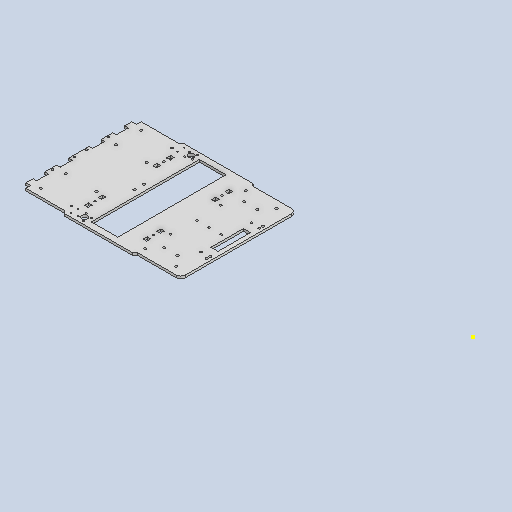
# Autodesk Inventor part: нижняя пластина
Saved by Autodesk Inventor 2024.2 (Build 282272000, 272)
## iProperties
Created: 2025-11-23
Part Number: нижняя пластина
Material: Типовые
Document SubType Name: Modeling
Designer: katya_notebook
Density: 1 g/cm^3
Appearance: По умолчанию
Author: katya_notebook
Autodesk Inventor part; units mm, degrees
ref_plane "YZ Plane" through (0, 0, 0) normal (1, 0, 0) x (0, 1, 0)
ref_plane "XZ Plane" through (0, 0, 0) normal (0, 1, 0) x (-1, 0, 0)
ref_plane "XY Plane" through (0, 0, 0) normal (0, 0, 1) x (1, 0, 0)
ref_plane "РабПлоскость1" through (-553.278877, -264.300199, 1.422232) normal (0, 1, 0) x (-1, 0, 0)
sketch "Эскиз1" plane through (-553.278877, -264.300199, 1.422232) normal (0, 1, 0) x (-1, 0, 0)
  line L0 (-30, 163.500004) -> (30, 163.500003)
  line L1 (-30, -31.5) -> (30, -31.5)
  line L2 (46.476267, 163.500003) -> (-223.523733, 163.500003)
  line L3 (-223.523733, 163.500003) -> (-223.523733, -31.5)
  line L4 (-223.523733, -31.5) -> (46.476267, -31.5)
  line L5 (46.476267, -31.5) -> (46.476267, 163.500003)
  point P0 (-553.278877, -1.422232)
  point P1 (-30, -30)
  point P2 (30, -30)
  point P3 (30, 162.000003)
  point P4 (-30, 162.000004)
  dimension "d1" = 270
  dimension "d6" = 0
  dimension "d7" = 0
  constraints: 8 end point, 2 coincident, 2 parallel, 1 horizontal, 1 perpendicular
  measures "d1" distance of L2.start L2.end
  measures "d6" distance from line of L4 L1.end
  measures "d7" distance from line of L2 L0.end
extrude "Выдавливание1" add sketch "Эскиз1" along normal blind 4
sketch "Эскиз2" plane through (-553.278877, -264.300199, 1.422232) normal (0, -1, 0) x (1, 0, 0)
  circle A0 centre (26, 108.500004) radius 2
  circle A1 centre (-26, 151.000003) radius 2
  circle A2 centre (26, 151.000004) radius 2
  circle A3 centre (-26, 108.500003) radius 2
  line L0 (-21.5, 122.000003) -> (-21.5, 157.000003)
  line L1 (-23.5, 122.000003) -> (-21.5, 122.000003)
  line L2 (-23.5, 157.000003) -> (-23.5, 122.000003)
  line L3 (-30, 157.000003) -> (-23.5, 157.000003)
  line L4 (-30, 157.000003) -> (-30, 103.500003)
  line L5 (-30, 103.500003) -> (30, 103.500004)
  line L6 (30, 103.500004) -> (30, 157.000004)
  line L7 (23.5, 157.000004) -> (30, 157.000004)
  line L8 (23.5, 122.000004) -> (23.5, 157.000004)
  line L9 (21.5, 122.000004) -> (23.5, 122.000004)
  line L10 (21.5, 157.000004) -> (21.5, 122.000004)
  line L11 (-21.5, 157.000003) -> (21.5, 157.000004)
  circle A4 centre (26, 23.5) radius 2
  circle A5 centre (-26, -19) radius 2
  circle A6 centre (26, -19) radius 2
  circle A7 centre (-26, 23.5) radius 2
  line L12 (-21.5, 10) -> (-21.5, -25)
  line L13 (-21.5, -25) -> (21.5, -25)
  line L14 (21.5, -25) -> (21.5, 10)
  line L15 (21.5, 10) -> (23.5, 10)
  line L16 (23.5, 10) -> (23.5, -25)
  line L17 (23.5, -25) -> (30, -25)
  line L18 (30, 28.5) -> (30, -25)
  line L19 (-30, 28.5) -> (30, 28.5)
  line L20 (-30, -25) -> (-30, 28.5)
  line L21 (-30, -25) -> (-23.5, -25)
  line L22 (-23.5, -25) -> (-23.5, 10)
  line L23 (-23.5, 10) -> (-21.5, 10)
  circle A8 centre (26, -19) radius 2
  circle A9 centre (26, 23.5) radius 2
  circle A10 centre (-26, -19) radius 2
  circle A11 centre (-26, 23.5) radius 2
  circle A12 centre (26, 108.500004) radius 2
  circle A13 centre (26, 151.000004) radius 2
  circle A14 centre (-26, 108.500003) radius 2
  circle A15 centre (-26, 151.000003) radius 2
  point P0 (553.278877, -1.422232)
  constraints: 8 centre point, 8 coincident, 8 concentric
extrude "Выдавливание2" cut sketch "Эскиз2" against normal blind 4 contours A0 | A1 | A2 | A3 | A4 | A5 | A6 | A7
sketch "Эскиз3" plane through (-553.278877, -264.300199, 1.422232) normal (0, -1, 0) x (1, 0, 0)
  spline S0 degree 3 poles (167.530647, -1.5) (167.530647, -1.675228) (167.505938, -1.863112) (167.406969, -2.216269) (167.332996, -2.381628) (167.143154, -2.701977) (167.002629, -2.869355) (166.694843, -3.139058) (166.528045, -3.241917) (165.99333, -3.490366) (165.589204, -3.533982) (164.848659, -3.417135) (164.512124, -3.257434) (164.024214, -2.845742) (163.799855, -2.568258) (163.628417, -2.126382) (163.592902, -2.011125) (163.543842, -1.762124) (163.530647, -1.627897) (163.530647, -1.372102) (163.543842, -1.237875) (163.592902, -0.988874) (163.628417, -0.873617) (163.799855, -0.431742) (164.024214, -0.154257) (164.512124, 0.257435) (164.848659, 0.417136) (165.589204, 0.533983) (165.99333, 0.490367) (166.528045, 0.241918) (166.694843, 0.139059) (167.002629, -0.130644) (167.143154, -0.298022) (167.332996, -0.618371) (167.406969, -0.78373) (167.505938, -1.136887) (167.530647, -1.324772) (167.530647, -1.5) knots -1.5971811 -1.5971811 -1.5971811 -1.5971811 -1.5446127 -1.5446127 -1.49204429 -1.49204429 -1.42257961 -1.42257961 -1.35311492 -1.35311492 -1.18239978 -1.18239978 -1.01168465 -1.01168465 -0.87532923 -0.87532923 -0.83695989 -0.83695989 -0.79859055 -0.79859055 -0.76022121 -0.76022121 -0.72185188 -0.72185188 -0.58549645 -0.58549645 -0.41478132 -0.41478132 -0.24406618 -0.24406618 -0.17460149 -0.17460149 -0.10513681 -0.10513681 -0.0525684 -0.0525684 0 0 0 0
  spline S1 degree 3 poles (190.047468, -1.5) (190.047468, -1.620288) (190.036518, -1.738724) (189.995823, -1.966144) (189.966063, -2.075131) (189.855778, -2.381563) (189.753425, -2.558671) (189.3863, -3.048352) (189.043184, -3.281704) (188.267032, -3.529213) (187.832995, -3.536652) (187.236348, -3.337829) (187.042108, -3.243447) (186.680736, -2.977295) (186.514082, -2.804962) (186.286366, -2.464282) (186.197167, -2.285548) (186.077558, -1.900195) (186.047468, -1.693486) (186.047468, -1.306513) (186.077558, -1.099804) (186.197167, -0.714451) (186.286366, -0.535718) (186.514082, -0.195037) (186.680736, -0.022705) (187.042108, 0.243448) (187.236348, 0.33783) (187.832995, 0.536653) (188.267032, 0.529214) (189.043184, 0.281704) (189.3863, 0.048353) (189.753425, -0.441328) (189.855778, -0.618437) (189.966063, -0.924868) (189.995823, -1.033855) (190.036518, -1.261275) (190.047468, -1.379712) (190.047468, -1.5) knots -1.53992103 -1.53992103 -1.53992103 -1.53992103 -1.50383465 -1.50383465 -1.46774826 -1.46774826 -1.39557548 -1.39557548 -1.21717391 -1.21717391 -1.03877234 -1.03877234 -0.96241242 -0.96241242 -0.88605249 -0.88605249 -0.8280065 -0.8280065 -0.76996052 -0.76996052 -0.71191453 -0.71191453 -0.65386854 -0.65386854 -0.57750862 -0.57750862 -0.50114869 -0.50114869 -0.32274712 -0.32274712 -0.14434556 -0.14434556 -0.07217278 -0.07217278 -0.03608639 -0.03608639 0 0 0 0
  circle A0 centre (203.047466, 23.5) radius 2
  circle A1 centre (203.047467, -19) radius 2
  circle A2 centre (151.047466, 23.5) radius 2
  circle A3 centre (151.047467, -19) radius 2
  line L0 (206.802962, 28.5) -> (146.802962, 28.5)
  line L1 (146.802962, 28.5) -> (146.802962, -22)
  line L2 (206.802962, -22) -> (206.802962, 28.5)
  line L3 (206.802962, -22) -> (146.802962, -22)
  point P0 (553.278877, -1.422232)
  point P1 (167.530647, -1.5)
  point P2 (190.047468, -1.5)
extrude "Выдавливание3" cut sketch "Эскиз3" against normal blind 10 contours S0 | S1 | A0 | A1 | A2 | A3
sketch "Эскиз4" plane through (-553.278877, -264.300199, 1.422232) normal (0, -1, 0) x (1, 0, 0)
  circle A0 centre (151.047466, 108.500004) radius 2
  circle A1 centre (203.047466, 108.500003) radius 2
  spline S0 degree 3 poles (190.047468, 133.500003) (190.047468, 133.620291) (190.036518, 133.738728) (189.995823, 133.966148) (189.966063, 134.075135) (189.855778, 134.381566) (189.753425, 134.558675) (189.3863, 135.048356) (189.043184, 135.281707) (188.267032, 135.529217) (187.832995, 135.536656) (187.236348, 135.337833) (187.042108, 135.243451) (186.680736, 134.977298) (186.514082, 134.804966) (186.286366, 134.464285) (186.197167, 134.285552) (186.077558, 133.900199) (186.047468, 133.69349) (186.047468, 133.306517) (186.077558, 133.099808) (186.197167, 132.714455) (186.286366, 132.535721) (186.514082, 132.195041) (186.680736, 132.022708) (187.042108, 131.756556) (187.236348, 131.662174) (187.832995, 131.46335) (188.267032, 131.47079) (189.043184, 131.718299) (189.3863, 131.95165) (189.753425, 132.441332) (189.855778, 132.61844) (189.966063, 132.924872) (189.995823, 133.033859) (190.036518, 133.261279) (190.047468, 133.379715) (190.047468, 133.500003) knots 0 0 0 0 0.03608639 0.03608639 0.07217278 0.07217278 0.14434556 0.14434556 0.32274712 0.32274712 0.50114869 0.50114869 0.57750862 0.57750862 0.65386854 0.65386854 0.71191453 0.71191453 0.76996052 0.76996052 0.8280065 0.8280065 0.88605249 0.88605249 0.96241242 0.96241242 1.03877234 1.03877234 1.21717391 1.21717391 1.39557548 1.39557548 1.46774826 1.46774826 1.50383465 1.50383465 1.53992103 1.53992103 1.53992103 1.53992103
  spline S1 degree 3 poles (167.530647, 133.500003) (167.530647, 133.675231) (167.505938, 133.863116) (167.406969, 134.216273) (167.332996, 134.381632) (167.143154, 134.701981) (167.002629, 134.869359) (166.694843, 135.139062) (166.528045, 135.241921) (165.99333, 135.49037) (165.589204, 135.533986) (164.848659, 135.417139) (164.512124, 135.257438) (164.024214, 134.845746) (163.799855, 134.568261) (163.628417, 134.126386) (163.592902, 134.011129) (163.543842, 133.762128) (163.530647, 133.627901) (163.530647, 133.372105) (163.543842, 133.237879) (163.592902, 132.988878) (163.628417, 132.873621) (163.799855, 132.431745) (164.024214, 132.154261) (164.512124, 131.742569) (164.848659, 131.582868) (165.589204, 131.466021) (165.99333, 131.509637) (166.528045, 131.758086) (166.694843, 131.860945) (167.002629, 132.130648) (167.143154, 132.298026) (167.332996, 132.618375) (167.406969, 132.783734) (167.505938, 133.136891) (167.530647, 133.324775) (167.530647, 133.500003) knots 0 0 0 0 0.0525684 0.0525684 0.10513681 0.10513681 0.17460149 0.17460149 0.24406618 0.24406618 0.41478132 0.41478132 0.58549645 0.58549645 0.72185188 0.72185188 0.76022121 0.76022121 0.79859055 0.79859055 0.83695989 0.83695989 0.87532923 0.87532923 1.01168465 1.01168465 1.18239978 1.18239978 1.35311492 1.35311492 1.42257961 1.42257961 1.49204429 1.49204429 1.5446127 1.5446127 1.5971811 1.5971811 1.5971811 1.5971811
  circle A2 centre (151.047467, 151.000004) radius 2
  circle A3 centre (203.047467, 151.000003) radius 2
  point P0 (553.278877, -1.422232)
  point P1 (190.047468, 133.500003)
  point P2 (167.530647, 133.500003)
extrude "Выдавливание4" cut sketch "Эскиз4" against normal blind 10
sketch "Эскиз6" plane through (-553.278877, -264.300199, 1.422232) normal (0, -1, 0) x (1, 0, 0)
  circle A0 centre (53.523733, 156.000002) radius 5
  circle A1 centre (53.523733, 156.000002) radius 2.5
  circle A2 centre (53.523733, 156.000002) radius 5
  circle A3 centre (53.523733, -23.999998) radius 5
  circle A4 centre (53.523733, -23.999998) radius 5
  point P0 (553.278877, -1.422232)
  constraints: 2 centre point, 2 coincident, 2 concentric
extrude "Выдавливание6" cut sketch "Эскиз6" against normal blind 10 contours A0 | A1 | A3
sketch "Эскиз7" plane through (-553.278877, -264.300199, 1.422232) normal (0, -1, 0) x (1, 0, 0)
  line L0 (30, 103.500004) -> (30, 157.000004)
  line L1 (-46.476267, 163.500003) -> (223.523733, 163.500003)
  line L2 (30.270127, 167.770131) -> (146.697322, 167.770131)
  line L3 (146.802962, 163.500003) -> (146.802962, 157.000003)
  line L4 (146.802962, 167.770131) -> (146.697322, 167.770131)
  line L5 (146.802962, 163.500003) -> (30, 163.500003)
  line L6 (30.000003, 28.5) -> (30.000003, -25)
  line L7 (30.000003, -25) -> (30.000003, -31.5)
  line L8 (146.802962, -31.5) -> (146.802962, -25)
  line L9 (146.802962, -35.5) -> (30.000003, -35.5)
  line L10 (30.000003, -31.5) -> (146.802962, -31.5)
  line L11 (30, 163.500003) -> (26, 163.500003)
  arc A0 (26, 163.500003) -> (30.270127, 167.770131) centre (22.8966, 170.873531) ccw
  line L12 (146.802962, 163.500003) -> (150.802962, 163.500003)
  arc A1 (146.802962, 167.770131) -> (150.802962, 163.500003) centre (154.237087, 170.72543) ccw
  line L13 (30.000003, -31.5) -> (26.000003, -31.5)
  line L14 (223.523733, -31.5) -> (-46.476267, -31.5)
  arc A2 (30.000003, -35.5) -> (26.000003, -31.5) centre (22.7085, -38.791502) ccw
  line L15 (146.802962, -31.5) -> (150.802962, -31.5)
  arc A3 (150.802962, -31.5) -> (146.802962, -35.5) centre (154.094465, -38.791502) ccw
  point P0 (553.278877, -1.422232)
  dimension "d23" = 8
  dimension "d24" = 8
  dimension "d26" = 8
  dimension "d28" = 8
  constraints: 18 end point, 8 point on circle, 5 point on line, 4 centre point, 2 collinear, 1 parallel
  measures "d23" radius of A0
  measures "d24" radius of A1
  measures "d26" radius of A2
  measures "d28" radius of A3
extrude "Выдавливание7" add sketch "Эскиз7" against normal blind 4
sketch "Эскиз8" plane through (-553.278877, -264.300199, 1.422232) normal (0, -1, 0) x (1, 0, 0)
  circle A0 centre (57.777238, 162.775524) radius 1.5
  circle A1 centre (60.299256, 151.746498) radius 1.5
  circle A2 centre (49.270229, 149.22448) radius 1.5
  circle A3 centre (46.748211, 160.253506) radius 1.5
  circle A4 centre (57.777238, 162.775524) radius 1.5
  circle A5 centre (60.299256, 151.746498) radius 1.5
  circle A6 centre (49.270229, 149.22448) radius 1.5
  circle A7 centre (46.748211, 160.253506) radius 1.5
  circle A8 centre (60.299256, -19.746494) radius 1.5
  circle A9 centre (57.777238, -30.775521) radius 1.5
  circle A10 centre (46.748211, -28.253503) radius 1.5
  circle A11 centre (49.270229, -17.224476) radius 1.5
  circle A12 centre (49.270229, -17.224476) radius 1.5
  circle A13 centre (60.299256, -19.746494) radius 1.5
  circle A14 centre (57.777238, -30.775521) radius 1.5
  circle A15 centre (46.748211, -28.253503) radius 1.5
  point P0 (553.278877, -1.422232)
  constraints: 8 centre point, 8 coincident, 8 concentric
extrude "Выдавливание8" cut sketch "Эскиз8" against normal blind 4
sketch "Эскиз9" plane through (-553.278877, -264.300199, 1.422232) normal (0, -1, 0) x (1, 0, 0)
  line L0 (223.523733, 163.500003) -> (223.523733, -31.5)
  line L1 (-46.476267, -31.5) -> (-46.476267, 163.500003)
  line L2 (223.523733, 163.500003) -> (-46.476267, 163.500003)
  line L3 (-46.476267, 163.500003) -> (-46.476267, -31.5)
  line L4 (-46.476267, -31.5) -> (223.523733, -31.5)
  line L5 (223.523733, -31.5) -> (223.523733, 163.500003)
  line L6 (223.523733, 66.000002) -> (-46.476267, 66.000002)
  line L7 (88.523733, 163.500003) -> (88.523733, -31.5)
  line L8 (66.023733, -25.499998) -> (111.023733, -25.499998)
  line L9 (111.023733, -25.499998) -> (111.023733, 157.500002)
  line L10 (111.023733, 157.500002) -> (66.023733, 157.500002)
  line L11 (66.023733, 157.500002) -> (66.023733, -25.499998)
  line L12 (66.023733, -25.499998) -> (111.023733, 157.500002) construction
  line L13 (111.023733, -25.499998) -> (66.023733, 157.500002) construction
  point P0 (553.278877, -1.422232)
  point P1 (88.523733, 66.000002)
  dimension "d33" = 183
  dimension "d34" = 45
  constraints: 24 end point, 7 midpoint, 4 parallel, 2 horizontal, 2 perpendicular
  measures "d33" distance of L8.end L9.end
  measures "d34" distance of L9.end L10.end
extrude "Выдавливание9" cut sketch "Эскиз9" against normal blind 4 contours L9 L8 L7 L6 | L6 L7 L10 L9 | L7 L6 L11 L10 | L7 L8 L11 L6
sketch "Эскиз10" plane through (-553.278877, -264.300199, 1.422232) normal (0, -1, 0) x (1, 0, 0)
  line L0 (36.973733, 147.850002) -> (34.973733, 147.850002)
  line L1 (36.973733, 147.850002) -> (36.973733, 152.650002)
  line L2 (35.973733, 147.850002) -> (35.973733, 152.650002)
  line L3 (36.973733, 159.350002) -> (34.973733, 159.350002)
  line L4 (36.973733, 150.250002) -> (34.973733, 150.250002)
  line L5 (36.973733, 159.350002) -> (36.973733, 164.150002)
  line L6 (36.973733, 161.750002) -> (33.994288, 161.750002)
  line L7 (33.994288, 161.750002) -> (35.973733, 159.350002)
  line L8 (35.973733, 164.150002) -> (35.973733, 159.350002)
  circle A0 centre (35.973733, 161.750002) radius 1
  circle A1 centre (35.973733, 150.250002) radius 1
  point P0 (553.278877, -1.422232)
  point P1 (34.973733, 147.000002)
  point P2 (30, 163.500005)
  point P3 (34.973733, 161.750002)
  point P4 (35.973733, 162.750002)
  point P5 (35.973733, 161.750002)
  constraints: 18 end point, 4 midpoint, 4 perpendicular, 2 horizontal, 1 horizontal alignment, 6 other
extrude "Выдавливание10" cut sketch "Эскиз10" against normal blind 10 contours A1 L2 L4 | L4 L2 A1 | A1 L4 L2 | L4 A1 L2 | A0 L8 L6 | L6 L8 A0 | A0 L6 L8 | L6 A0 L8
sketch "Эскиз11" plane through (-553.278877, -264.300199, 1.422232) normal (0, -1, 0) x (1, 0, 0)
  arc A0 (34.973733, -29.749998) -> (36.973733, -29.749998) centre (35.973733, -29.749998) ccw
  arc A1 (36.973733, -29.749998) -> (34.973733, -29.749998) centre (35.973733, -29.749998) ccw
  arc A2 (34.973733, -18.249998) -> (36.973733, -18.249998) centre (35.973733, -18.249998) ccw
  arc A3 (36.973733, -18.249998) -> (34.973733, -18.249998) centre (35.973733, -18.249998) ccw
  point P0 (553.278877, -1.422232)
extrude "Выдавливание11" cut sketch "Эскиз11" against normal blind 10
sketch "Эскиз12" plane through (-553.278877, -264.300199, 1.422232) normal (0, -1, 0) x (1, 0, 0)
  circle A0 centre (55.548733, 57.85394) radius 2
  circle A1 centre (55.548733, 73.85394) radius 2
  point P0 (553.278877, -1.422232)
extrude "Выдавливание12" cut sketch "Эскиз12" against normal blind 10
sketch "Эскиз13" plane through (-553.278877, -264.300199, 1.422232) normal (0, -1, 0) x (1, 0, 0)
  point P0 (553.278877, -1.422232)
sketch "Эскиз14" plane through (-553.278877, -264.300199, 1.422232) normal (0, -1, 0) x (1, 0, 0)
  circle A0 centre (217.523733, 18.5) radius 2
  circle A1 centre (217.523733, 113.500003) radius 2
  line L0 (150.802962, 163.500003) -> (223.523733, 163.500003)
  line L1 (223.523733, -31.5) -> (150.802962, -31.5)
  line L2 (223.523733, 163.500003) -> (223.523733, -31.5)
  circle A2 centre (217.523733, 24.5) radius 2
  circle A3 centre (217.523733, 107.500003) radius 2
  point P0 (553.278877, -1.422232)
  dimension "d43" = 4
  dimension "d44" = 4
  dimension "d45" = 50
  dimension "d46" = 50
  dimension "d47" = 6
  dimension "d48" = 6
  dimension "d51" = 4
  dimension "d52" = 6
  dimension "d53" = 6
  dimension "d54" = 4
  dimension "d55" = 6
  dimension "d56" = 6
  constraints: 4 centre point
  measures "d43" diameter of A1
  measures "d44" diameter of A0
  measures "d45" distance from line of L0 A1.centre
  measures "d46" distance from line of L1 A0.centre
  measures "d47" distance from line of L2 A0.centre
  measures "d48" distance from line of L2 A1.centre
  measures "d51" diameter of A3
  measures "d52" distance of A1.centre A3.centre
  measures "d53" distance from line of L2 A3.centre
  measures "d54" diameter of A2
  measures "d55" distance from line of L2 A2.centre
  measures "d56" distance of A0.centre A2.centre
extrude "Выдавливание13" cut sketch "Эскиз14" against normal blind 10
sketch "Эскиз15" plane through (-553.278877, -264.300199, 1.422232) normal (0, -1, 0) x (1, 0, 0)
  line L0 (216.523733, 93.576493) -> (204.523733, 93.576493)
  line L1 (204.523733, 93.576493) -> (204.523733, 38.576493)
  line L2 (204.523733, 38.576493) -> (216.523733, 38.576493)
  line L3 (216.523733, 38.576493) -> (216.523733, 93.576493)
  line L4 (216.523733, 93.576493) -> (204.523733, 38.576493) construction
  line L5 (204.523733, 93.576493) -> (216.523733, 38.576493) construction
  line L6 (223.523733, 163.500003) -> (223.523733, -31.5)
  point P0 (553.278877, -1.422232)
  point P1 (210.523733, 66.076493)
  dimension "d57" = 13
  dimension "d58" = 12
  dimension "d59" = 55
  constraints: 12 end point, 2 midpoint, 2 parallel, 1 horizontal, 1 perpendicular
  measures "d57" distance from line of point (210.524, 66.076) L6
  measures "d58" distance of L0.start L0.end
  measures "d59" distance of L0.end L1.end
extrude "Выдавливание14" cut sketch "Эскиз15" against normal blind 10
sketch "Эскиз16" plane through (-553.278877, -264.300199, 1.422232) normal (0, -1, 0) x (1, 0, 0)
  spline S0 degree 3 poles (195.773733, 65.9) (195.773733, 66.088725) (195.735944, 66.289784) (195.582756, 66.659245) (195.467375, 66.827679) (195.201416, 67.093638) (195.03298, 67.209022) (194.663513, 67.362213) (194.462453, 67.4) (194.085014, 67.4) (193.883953, 67.362213) (193.514486, 67.209022) (193.346051, 67.093638) (193.080092, 66.827679) (192.964711, 66.659245) (192.811522, 66.289784) (192.773733, 66.088725) (192.773733, 65.711276) (192.811522, 65.510217) (192.964711, 65.140756) (193.080092, 64.972321) (193.346051, 64.706363) (193.514486, 64.590979) (193.883953, 64.437788) (194.085014, 64.4) (194.462453, 64.4) (194.663513, 64.437788) (195.03298, 64.590979) (195.201416, 64.706363) (195.467375, 64.972321) (195.582756, 65.140756) (195.735944, 65.510217) (195.773733, 65.711276) (195.773733, 65.9) knots -0.905867 -0.905867 -0.905867 -0.905867 -0.84924956 -0.84924956 -0.79263212 -0.79263212 -0.73601619 -0.73601619 -0.67940025 -0.67940025 -0.62278432 -0.62278432 -0.56616839 -0.56616839 -0.50955095 -0.50955095 -0.4529335 -0.4529335 -0.39631606 -0.39631606 -0.33969861 -0.33969861 -0.28308268 -0.28308268 -0.22646675 -0.22646675 -0.16985082 -0.16985082 -0.11323489 -0.11323489 -0.05661744 -0.05661744 0 0 0 0
  spline S1 degree 3 poles (172.273733, 66.1) (172.273733, 65.911276) (172.311522, 65.710217) (172.464711, 65.340756) (172.580092, 65.172321) (172.846051, 64.906363) (173.014486, 64.790979) (173.383953, 64.637788) (173.585014, 64.6) (173.962453, 64.6) (174.163513, 64.637788) (174.53298, 64.790979) (174.701416, 64.906363) (174.967375, 65.172321) (175.082756, 65.340756) (175.235944, 65.710217) (175.273733, 65.911276) (175.273733, 66.288725) (175.235944, 66.489784) (175.082756, 66.859245) (174.967375, 67.027679) (174.701416, 67.293638) (174.53298, 67.409022) (174.163513, 67.562213) (173.962453, 67.6) (173.585014, 67.6) (173.383953, 67.562213) (173.014486, 67.409022) (172.846051, 67.293638) (172.580092, 67.027679) (172.464711, 66.859245) (172.311522, 66.489784) (172.273733, 66.288725) (172.273733, 66.1) knots -0.905867 -0.905867 -0.905867 -0.905867 -0.84924956 -0.84924956 -0.79263212 -0.79263212 -0.73601619 -0.73601619 -0.67940025 -0.67940025 -0.62278432 -0.62278432 -0.56616839 -0.56616839 -0.50955095 -0.50955095 -0.4529335 -0.4529335 -0.39631606 -0.39631606 -0.33969861 -0.33969861 -0.28308268 -0.28308268 -0.22646675 -0.22646675 -0.16985082 -0.16985082 -0.11323489 -0.11323489 -0.05661744 -0.05661744 0 0 0 0
  spline S2 degree 3 poles (154.773733, 65.9) (154.773733, 66.088725) (154.735944, 66.289784) (154.582756, 66.659245) (154.467375, 66.827679) (154.201416, 67.093638) (154.03298, 67.209022) (153.663513, 67.362213) (153.462453, 67.4) (153.085014, 67.4) (152.883953, 67.362213) (152.514486, 67.209022) (152.346051, 67.093638) (152.080092, 66.827679) (151.964711, 66.659245) (151.811522, 66.289784) (151.773733, 66.088725) (151.773733, 65.711276) (151.811522, 65.510217) (151.964711, 65.140756) (152.080092, 64.972321) (152.346051, 64.706363) (152.514486, 64.590979) (152.883953, 64.437788) (153.085014, 64.4) (153.462453, 64.4) (153.663513, 64.437788) (154.03298, 64.590979) (154.201416, 64.706363) (154.467375, 64.972321) (154.582756, 65.140756) (154.735944, 65.510217) (154.773733, 65.711276) (154.773733, 65.9) knots -0.905867 -0.905867 -0.905867 -0.905867 -0.84924956 -0.84924956 -0.79263212 -0.79263212 -0.73601619 -0.73601619 -0.67940025 -0.67940025 -0.62278432 -0.62278432 -0.56616839 -0.56616839 -0.50955095 -0.50955095 -0.4529335 -0.4529335 -0.39631606 -0.39631606 -0.33969861 -0.33969861 -0.28308268 -0.28308268 -0.22646675 -0.22646675 -0.16985082 -0.16985082 -0.11323489 -0.11323489 -0.05661744 -0.05661744 0 0 0 0
  point P0 (553.278877, -1.422232)
  point P1 (195.773733, 65.9)
  point P2 (172.273733, 66.1)
  point P3 (154.773733, 65.9)
extrude "Выдавливание15" cut sketch "Эскиз16" against normal blind 10
sketch "Эскиз17" plane through (-553.278877, -260.300199, 1.422232) normal (0, 1, 0) x (1, 0, 0)
  line L0 (-46.476267, -143.500003) -> (-46.476267, -123.500003)
  line L1 (-46.476267, -143.500003) -> (-40.476267, -143.500003)
  line L2 (-40.476267, -123.500003) -> (-40.476267, -143.500003)
  line L3 (-46.476267, -123.500003) -> (-40.476267, -123.500003)
  line L4 (-46.476267, -103.500003) -> (-46.476267, -83.500003)
  line L5 (-46.476267, -103.500003) -> (-40.476267, -103.500003)
  line L6 (-40.476267, -83.500003) -> (-40.476267, -103.500003)
  line L7 (-46.476267, -83.500003) -> (-40.476267, -83.500003)
  line L8 (-46.476267, -48.5) -> (-46.476267, -28.5)
  line L9 (-46.476267, -48.5) -> (-40.476267, -48.5)
  line L10 (-40.476267, -28.5) -> (-40.476267, -48.5)
  line L11 (-46.476267, -28.5) -> (-40.476267, -28.5)
  line L12 (-46.476267, -8.5) -> (-46.476267, 11.5)
  line L13 (-46.476267, -8.5) -> (-40.476267, -8.5)
  line L14 (-40.476267, 11.5) -> (-40.476267, -8.5)
  line L15 (-46.476267, 11.5) -> (-40.476267, 11.5)
  circle A0 centre (-43.476267, -113.500003) radius 1.75
  circle A1 centre (-43.476267, -76.375003) radius 1.75
  circle A2 centre (-43.476267, -55.625003) radius 1.75
  circle A3 centre (-43.476267, -18.5) radius 1.75
  point P0 (553.278877, 1.422232)
extrude "Выдавливание16" cut sketch "Эскиз17" against normal blind 10
fillet "Сопряжение1" radius 8 4 edges at (-329.7551, -262.3002, -30.0778) (-329.7551, -262.3002, 164.9222) (-599.7551, -262.3002, -30.0778) (-599.7551, -262.3002, 164.9222)
sketch "Эскиз18" plane through (-599.755143, -264.300199, 104.922235) normal (-1, 0, 0) x (0, 0, 1)
  line L0 (-95.000003, 0) -> (-95.000003, 4)
  line L1 (-95.000003, 4) -> (-95.000003, 5)
  line L2 (-95.000003, 5) -> (-115.000003, 5)
  line L3 (-115.000003, 5) -> (-115.000003, 4)
  line L4 (-135.000003, 4) -> (-127.000003, 4)
  line L5 (-135.000003, 4) -> (-135.000003, -55.704973)
  line L6 (-115.000003, -55.704973) -> (-135.000003, -55.704973)
  line L7 (-115.000003, -55.704973) -> (-115.000003, -60.704973)
  line L8 (-115.000003, -60.704973) -> (-95.000003, -60.704973)
  line L9 (-95.000003, -60.704973) -> (-95.000003, -55.704973)
  line L10 (-86.750003, -55.704973) -> (-95.000003, -55.704973)
  line L11 (-86.750003, -55.704973) -> (-86.750003, -54.204972)
  line L12 (-86.750003, -54.204972) -> (-88.250003, -54.204972)
  line L13 (-88.250003, -54.204972) -> (-88.250003, -51.204972)
  line L14 (-88.250003, -51.204972) -> (-86.750003, -51.204972)
  line L15 (-86.750003, -51.204972) -> (-86.750003, -43.704972)
  line L16 (-86.750003, -43.704972) -> (-83.250003, -43.704972)
  line L17 (-83.250003, -43.704972) -> (-83.250003, -51.204972)
  line L18 (-83.250003, -51.204972) -> (-81.750003, -51.204972)
  line L19 (-81.750003, -51.204972) -> (-81.750003, -54.204972)
  line L20 (-81.750003, -54.204972) -> (-83.250003, -54.204972)
  line L21 (-83.250003, -54.204972) -> (-83.250003, -55.704973)
  line L22 (-75.000003, -55.704973) -> (-83.250003, -55.704973)
  line L23 (-75.000003, -55.704973) -> (-75.000003, -60.704973)
  line L24 (-75.000003, -60.704973) -> (-55.000003, -60.704972)
  line L25 (-55.000003, -60.704972) -> (-55.000003, -55.704972)
  line L26 (-49.624972, -55.704972) -> (-55.000003, -55.704972)
  line L27 (-49.624972, -55.704972) -> (-49.624972, -54.204972)
  line L28 (-49.624972, -54.204972) -> (-51.124972, -54.204972)
  line L29 (-51.124972, -54.204972) -> (-51.124972, -51.204972)
  line L30 (-51.124972, -51.204972) -> (-49.624972, -51.204972)
  line L31 (-49.624972, -51.204972) -> (-49.624972, -49.704972)
  line L32 (-49.624972, -49.704972) -> (-49.625, -49.704972)
  line L33 (-49.625, -49.704972) -> (-49.625, -43.704972)
  line L34 (-49.625, -43.704972) -> (-46.124972, -43.704972)
  line L35 (-46.124972, -43.704972) -> (-46.124972, -51.204972)
  line L36 (-46.124972, -51.204972) -> (-44.624972, -51.204972)
  line L37 (-44.624972, -51.204972) -> (-44.624972, -54.204972)
  line L38 (-44.624972, -54.204972) -> (-46.124972, -54.204972)
  line L39 (-46.124972, -54.204972) -> (-46.124972, -55.704972)
  line L40 (-28.875, -55.704972) -> (-46.124972, -55.704972)
  line L41 (-28.875, -55.704972) -> (-28.875, -54.204972)
  line L42 (-28.875, -54.204972) -> (-30.375, -54.204972)
  line L43 (-30.375, -54.204972) -> (-30.375, -51.204972)
  line L44 (-30.375, -51.204972) -> (-28.875, -51.204972)
  line L45 (-28.875, -51.204972) -> (-28.875, -43.704972)
  line L46 (-28.875, -43.704972) -> (-25.375, -43.704972)
  line L47 (-25.375, -43.704972) -> (-25.375, -51.204972)
  line L48 (-25.375, -51.204972) -> (-23.875, -51.204972)
  line L49 (-23.875, -51.204972) -> (-23.875, -54.204972)
  line L50 (-23.875, -54.204972) -> (-25.375, -54.204972)
  line L51 (-25.375, -54.204972) -> (-25.375, -55.704972)
  line L52 (-20, -55.704972) -> (-25.375, -55.704972)
  line L53 (-20, -55.704972) -> (-20, -60.704972)
  line L54 (-20, -60.704972) -> (0, -60.704972)
  line L55 (0, -60.704972) -> (0, -55.704972)
  line L56 (8.25, -55.704972) -> (0, -55.704972)
  line L57 (8.25, -55.704972) -> (8.25, -54.204972)
  line L58 (8.25, -54.204972) -> (6.75, -54.204972)
  line L59 (6.75, -54.204972) -> (6.75, -51.204972)
  line L60 (6.75, -51.204972) -> (8.25, -51.204972)
  line L61 (8.25, -51.204972) -> (8.25, -43.704972)
  line L62 (8.25, -43.704972) -> (11.75, -43.704972)
  line L63 (11.75, -43.704972) -> (11.75, -51.204972)
  line L64 (11.75, -51.204972) -> (13.25, -51.204972)
  line L65 (13.25, -51.204972) -> (13.25, -54.204972)
  line L66 (13.25, -54.204972) -> (11.75, -54.204972)
  line L67 (11.75, -54.204972) -> (11.75, -55.704972)
  line L68 (20, -55.704972) -> (11.75, -55.704972)
  line L69 (20, -55.704972) -> (20, -60.704972)
  line L70 (20, -60.704972) -> (40, -60.704972)
  line L71 (40, -60.704972) -> (40, -55.704972)
  line L72 (60, -55.704972) -> (40, -55.704972)
  line L73 (60, 4) -> (60, -55.704972)
  line L74 (52, 4) -> (60, 4)
  line L75 (40, 4) -> (40, 5)
  line L76 (40, 5) -> (20, 5)
  line L77 (20, 5) -> (20, 4)
  line L78 (20, 4) -> (20, 0)
  line L79 (20, 0) -> (13.25, 0)
  line L80 (13.25, 0) -> (13.25, -0.5)
  line L81 (13.25, -0.5) -> (11.75, -0.5)
  line L82 (11.75, -0.5) -> (11.75, -8)
  line L83 (11.75, -8) -> (8.25, -8)
  line L84 (8.25, -8) -> (8.25, -0.5)
  line L85 (8.25, -0.5) -> (6.75, -0.5)
  line L86 (6.75, -0.5) -> (6.75, 0)
  line L87 (6.75, 0) -> (0, 0)
  line L88 (0, 0) -> (0, 4)
  line L89 (0, 4) -> (0, 5)
  line L90 (0, 5) -> (-20, 5)
  line L91 (-20, 5) -> (-20, 4)
  line L92 (-20, 4) -> (-20, 0)
  line L93 (-20, 0) -> (-23.875, 0)
  line L94 (-23.875, 0) -> (-23.875, -0.5)
  line L95 (-23.875, -0.5) -> (-25.375, -0.5)
  line L96 (-25.375, -0.5) -> (-25.375, -8)
  line L97 (-25.375, -8) -> (-28.875, -8)
  line L98 (-28.875, -8) -> (-28.875, -0.5)
  line L99 (-28.875, -0.5) -> (-30.375, -0.5)
  line L100 (-30.375, -0.5) -> (-30.375, 0)
  line L101 (-30.375, 0) -> (-44.624972, 0)
  line L102 (-44.624972, 0) -> (-44.624972, -0.5)
  line L103 (-44.624972, -0.5) -> (-46.124972, -0.5)
  line L104 (-46.124972, -0.5) -> (-46.124972, -8)
  line L105 (-46.124972, -8) -> (-49.625, -8)
  line L106 (-49.625, -8) -> (-49.625, -2)
  line L107 (-49.625, -2) -> (-49.624972, -2)
  line L108 (-49.624972, -2) -> (-49.624972, -0.5)
  line L109 (-49.624972, -0.5) -> (-51.124972, -0.5)
  line L110 (-51.124972, -0.5) -> (-51.124972, 0)
  line L111 (-51.124972, 0) -> (-55.000003, 0)
  line L112 (-55.000003, 0) -> (-55.000003, 4)
  line L113 (-55.000003, 4) -> (-55.000003, 5)
  line L114 (-55.000003, 5) -> (-75.000003, 5)
  line L115 (-75.000003, 5) -> (-75.000003, 4)
  line L116 (-75.000003, 4) -> (-75.000003, 0)
  line L117 (-75.000003, 0) -> (-81.750003, 0)
  line L118 (-81.750003, 0) -> (-81.750003, -0.5)
  line L119 (-81.750003, -0.5) -> (-83.250003, -0.5)
  line L120 (-83.250003, -0.5) -> (-83.250003, -8)
  line L121 (-83.250003, -8) -> (-86.750003, -8)
  line L122 (-86.750003, -8) -> (-86.750003, -0.5)
  line L123 (-86.750003, -0.5) -> (-88.250003, -0.5)
  line L124 (-88.250003, -0.5) -> (-88.250003, 0)
  line L125 (-88.250003, 0) -> (-95.000003, 0)
  line L126 (52, 0) -> (-127.000003, 0)
  line L127 (52, 0) -> (52, 4)
  line L128 (52, 4) -> (60, 4)
  line L129 (60, 0) -> (60, 4)
  line L130 (60, 0) -> (52, 0)
  line L131 (-127.000003, 0) -> (-127.000003, 4)
  line L132 (-135.000003, 0) -> (-135.000003, 4)
  line L133 (-127.000003, 4) -> (-135.000003, 4)
  line L134 (-135.000003, 0) -> (-127.000003, 0)
  line L135 (-127.000003, 0) -> (-127.000003, 4)
  line L136 (52, 4) -> (52, 0)
  line L137 (52, 0) -> (40, 0)
  line L138 (40, 0) -> (40, 4)
  line L139 (-115.000003, 4) -> (-115.000003, 0)
  line L140 (-115.000003, 0) -> (-127.000003, 0)
  point P0 (-104.922236, 264.300199)
  constraints: 16 end point, 6 perpendicular, 4 point on line, 2 parallel, 1 other
extrude "Выдавливание17" cut sketch "Эскиз18" against normal blind 8 contours L134 L5 L4 L131 | L127 L74 L73 L130
sketch "Эскиз19" plane through (-553.278877, -264.300199, 1.422232) normal (0, -1, 0) x (1, 0, 0)
  line L0 (41.9631, 0.000002) -> (41.9631, -6.999998)
  line L1 (41.9631, 0.000002) -> (35.9631, 0.000002)
  line L2 (35.9631, -6.999998) -> (35.9631, 0.000002)
  line L3 (41.9631, -6.999998) -> (35.9631, -6.999998)
  circle A0 centre (38.9631, 8.000002) radius 1.75
  line L4 (41.9631, 23.000002) -> (41.9631, 16.000002)
  line L5 (41.9631, 23.000002) -> (35.9631, 23.000002)
  line L6 (35.9631, 16.000002) -> (35.9631, 23.000002)
  line L7 (41.9631, 16.000002) -> (35.9631, 16.000002)
  line L8 (490.372561, 65.867736) -> (-34.635408, 65.867736)
  line L9 (35.9631, 109.000001) -> (35.9631, 116.000001)
  line L10 (41.9631, 109.000001) -> (35.9631, 109.000001)
  line L11 (41.9631, 116.000001) -> (41.9631, 109.000001)
  line L12 (35.9631, 116.000001) -> (41.9631, 116.000001)
  circle A1 centre (38.9631, 124.000001) radius 1.75
  line L13 (41.9631, 132.000001) -> (35.9631, 132.000001)
  line L14 (35.9631, 132.000001) -> (35.9631, 139.000001)
  line L15 (35.9631, 139.000001) -> (41.9631, 139.000001)
  line L16 (41.9631, 139.000001) -> (41.9631, 132.000001)
  line L17 (135.084367, 0.000002) -> (141.084367, 0.000002)
  line L18 (135.084367, -6.999998) -> (135.084367, 0.000002)
  line L19 (135.324736, -6.999997) -> (136.629737, -6.999997)
  line L20 (141.084367, -6.999998) -> (135.084367, -6.999998)
  line L21 (141.084367, 0.000002) -> (141.084367, -6.999998)
  line L22 (135.084367, 16.000002) -> (135.084367, 23.000002)
  line L23 (141.084367, 16.000002) -> (135.084367, 16.000002)
  line L24 (141.084367, 23.000002) -> (141.084367, 16.000002)
  line L25 (135.084367, 23.000002) -> (141.084367, 23.000002)
  circle A2 centre (138.084367, 8.000002) radius 1.75
  line L26 (135.084367, 109.000001) -> (135.084367, 116.000001)
  line L27 (135.084367, 116.000001) -> (141.084367, 116.000001)
  line L28 (141.084367, 109.000001) -> (135.084367, 109.000001)
  line L29 (141.084367, 116.000001) -> (141.084367, 109.000001)
  circle A3 centre (138.383276, 122.178003) radius 0.9
  circle A4 centre (138.084367, 124.000001) radius 1.75
  line L30 (188.226871, 146.409) -> (188.226871, 95.659004)
  line L31 (188.226871, 95.659004) -> (164.226871, 95.659004)
  line L32 (164.226871, 95.659004) -> (164.226871, 146.409)
  line L33 (164.226871, 146.409) -> (188.226871, 146.409)
  line L34 (141.084367, 23.000002) -> (141.084367, 16.000002)
  line L35 (141.084367, 16.000002) -> (135.084367, 16.000002)
  line L36 (135.084367, 16.000002) -> (135.084367, 23.000002)
  line L37 (135.084367, 23.000002) -> (141.084367, 23.000002)
  line L38 (35.9631, 132.000001) -> (35.9631, 139.000001)
  line L39 (35.9631, 139.000001) -> (41.9631, 139.000001)
  line L40 (41.9631, 139.000001) -> (41.9631, 132.000001)
  line L41 (41.9631, 132.000001) -> (35.9631, 132.000001)
  circle A5 centre (38.9631, 8.000002) radius 1.75
  line L42 (41.9631, -6.999998) -> (35.9631, -6.999998)
  line L43 (35.9631, -6.999998) -> (35.9631, 0.000002)
  line L44 (35.9631, 0.000002) -> (41.9631, 0.000002)
  line L45 (41.9631, 0.000002) -> (41.9631, -6.999998)
  line L46 (141.084367, 139.000001) -> (141.084367, 132.000001)
  line L47 (141.084367, 132.000001) -> (135.084367, 132.000001)
  line L48 (135.084367, 132.000001) -> (135.084367, 139.000001)
  line L49 (135.084367, 139.000001) -> (141.084367, 139.000001)
  circle A6 centre (138.084367, 8.000002) radius 1.75
  line L50 (141.084367, 116.000001) -> (141.084367, 109.000001)
  line L51 (141.084367, 109.000001) -> (135.084367, 109.000001)
  line L52 (135.084367, 109.000001) -> (135.084367, 116.000001)
  line L53 (135.084367, 116.000001) -> (141.084367, 116.000001)
  circle A7 centre (38.9631, 124.000001) radius 1.75
  line L54 (41.9631, 16.000002) -> (35.9631, 16.000002)
  line L55 (35.9631, 16.000002) -> (35.9631, 23.000002)
  line L56 (35.9631, 23.000002) -> (41.9631, 23.000002)
  line L57 (41.9631, 23.000002) -> (41.9631, 16.000002)
  line L58 (35.9631, 109.000001) -> (35.9631, 116.000001)
  line L59 (35.9631, 116.000001) -> (41.9631, 116.000001)
  line L60 (41.9631, 116.000001) -> (41.9631, 109.000001)
  line L61 (41.9631, 109.000001) -> (35.9631, 109.000001)
  circle A8 centre (138.084367, 124.000001) radius 1.75
  line L62 (141.084367, 0.000002) -> (141.084367, -6.999998)
  line L63 (141.084367, -6.999998) -> (135.084367, -6.999998)
  line L64 (135.084367, -6.999998) -> (135.084367, 0.000002)
  line L65 (135.084367, 0.000002) -> (141.084367, 0.000002)
  circle A9 centre (130.911055, -16.502322) radius 1.285924
  circle A10 centre (209.546122, 19.017578) radius 1.300502
  circle A11 centre (130.955192, 19.034498) radius 1.251606
  circle A12 centre (209.490361, -16.508496) radius 1.341374
  circle A13 centre (194.523733, 85.500003) radius 1.6
  spline S0 degree 3 poles (38.773733, 66.100003) (38.773733, 66.288728) (38.811522, 66.489786) (38.964711, 66.859248) (39.080092, 67.027682) (39.346051, 67.293641) (39.514486, 67.409025) (39.883953, 67.562215) (40.085014, 67.600003) (40.462453, 67.600003) (40.663513, 67.562215) (41.03298, 67.409025) (41.201416, 67.293641) (41.467375, 67.027682) (41.582756, 66.859248) (41.735944, 66.489786) (41.773733, 66.288728) (41.773733, 65.911278) (41.735944, 65.71022) (41.582756, 65.340758) (41.467375, 65.172324) (41.201416, 64.906365) (41.03298, 64.790982) (40.663513, 64.637791) (40.462453, 64.600003) (40.085014, 64.600003) (39.883953, 64.637791) (39.514486, 64.790982) (39.346051, 64.906365) (39.080092, 65.172324) (38.964711, 65.340758) (38.811522, 65.71022) (38.773733, 65.911278) (38.773733, 66.100003) knots 0 0 0 0 0.05661744 0.05661744 0.11323489 0.11323489 0.16985082 0.16985082 0.22646675 0.22646675 0.28308268 0.28308268 0.33969861 0.33969861 0.39631606 0.39631606 0.4529335 0.4529335 0.50955095 0.50955095 0.56616839 0.56616839 0.62278432 0.62278432 0.67940025 0.67940025 0.73601619 0.73601619 0.79263212 0.79263212 0.84924956 0.84924956 0.905867 0.905867 0.905867 0.905867
  spline S1 degree 3 poles (-19.726267, 65.900003) (-19.726267, 65.711278) (-19.764056, 65.51022) (-19.917244, 65.140758) (-20.032625, 64.972324) (-20.298584, 64.706365) (-20.46702, 64.590982) (-20.836487, 64.437791) (-21.037547, 64.400003) (-21.414986, 64.400003) (-21.616047, 64.437791) (-21.985514, 64.590982) (-22.153949, 64.706365) (-22.419908, 64.972324) (-22.535289, 65.140758) (-22.688478, 65.51022) (-22.726267, 65.711278) (-22.726267, 66.088728) (-22.688478, 66.289786) (-22.535289, 66.659248) (-22.419908, 66.827682) (-22.153949, 67.093641) (-21.985514, 67.209025) (-21.616047, 67.362215) (-21.414986, 67.400003) (-21.037547, 67.400003) (-20.836487, 67.362215) (-20.46702, 67.209025) (-20.298584, 67.093641) (-20.032625, 66.827682) (-19.917244, 66.659248) (-19.764056, 66.289786) (-19.726267, 66.088728) (-19.726267, 65.900003) knots 0 0 0 0 0.05661744 0.05661744 0.11323489 0.11323489 0.16985082 0.16985082 0.22646675 0.22646675 0.28308268 0.28308268 0.33969861 0.33969861 0.39631606 0.39631606 0.4529335 0.4529335 0.50955095 0.50955095 0.56616839 0.56616839 0.62278432 0.62278432 0.67940025 0.67940025 0.73601619 0.73601619 0.79263212 0.79263212 0.84924956 0.84924956 0.905867 0.905867 0.905867 0.905867
  circle A14 centre (132.523733, 149.500003) radius 1.6
  circle A15 centre (132.523733, 37.500003) radius 1.6
  circle A16 centre (132.523733, 85.500003) radius 1.6
  spline S2 degree 3 poles (21.273733, 65.900003) (21.273733, 65.711278) (21.235944, 65.51022) (21.082756, 65.140758) (20.967375, 64.972324) (20.701416, 64.706365) (20.53298, 64.590982) (20.163513, 64.437791) (19.962453, 64.400003) (19.585014, 64.400003) (19.383953, 64.437791) (19.014486, 64.590982) (18.846051, 64.706365) (18.580092, 64.972324) (18.464711, 65.140758) (18.311522, 65.51022) (18.273733, 65.711278) (18.273733, 66.088728) (18.311522, 66.289786) (18.464711, 66.659248) (18.580092, 66.827682) (18.846051, 67.093641) (19.014486, 67.209025) (19.383953, 67.362215) (19.585014, 67.400003) (19.962453, 67.400003) (20.163513, 67.362215) (20.53298, 67.209025) (20.701416, 67.093641) (20.967375, 66.827682) (21.082756, 66.659248) (21.235944, 66.289786) (21.273733, 66.088728) (21.273733, 65.900003) knots 0 0 0 0 0.05661744 0.05661744 0.11323489 0.11323489 0.16985082 0.16985082 0.22646675 0.22646675 0.28308268 0.28308268 0.33969861 0.33969861 0.39631606 0.39631606 0.4529335 0.4529335 0.50955095 0.50955095 0.56616839 0.56616839 0.62278432 0.62278432 0.67940025 0.67940025 0.73601619 0.73601619 0.79263212 0.79263212 0.84924956 0.84924956 0.905867 0.905867 0.905867 0.905867
  spline S3 degree 3 poles (-2.226267, 66.100003) (-2.226267, 66.288728) (-2.188478, 66.489786) (-2.035289, 66.859248) (-1.919908, 67.027682) (-1.653949, 67.293641) (-1.485514, 67.409025) (-1.116047, 67.562215) (-0.914986, 67.600003) (-0.537547, 67.600003) (-0.336487, 67.562215) (0.03298, 67.409025) (0.201416, 67.293641) (0.467375, 67.027682) (0.582756, 66.859248) (0.735944, 66.489786) (0.773733, 66.288728) (0.773733, 65.911278) (0.735944, 65.71022) (0.582756, 65.340758) (0.467375, 65.172324) (0.201416, 64.906365) (0.03298, 64.790982) (-0.336487, 64.637791) (-0.537547, 64.600003) (-0.914986, 64.600003) (-1.116047, 64.637791) (-1.485514, 64.790982) (-1.653949, 64.906365) (-1.919908, 65.172324) (-2.035289, 65.340758) (-2.188478, 65.71022) (-2.226267, 65.911278) (-2.226267, 66.100003) knots 0 0 0 0 0.05661744 0.05661744 0.11323489 0.11323489 0.16985082 0.16985082 0.22646675 0.22646675 0.28308268 0.28308268 0.33969861 0.33969861 0.39631606 0.39631606 0.4529335 0.4529335 0.50955095 0.50955095 0.56616839 0.56616839 0.62278432 0.62278432 0.67940025 0.67940025 0.73601619 0.73601619 0.79263212 0.79263212 0.84924956 0.84924956 0.905867 0.905867 0.905867 0.905867
  circle A17 centre (194.523733, 149.500003) radius 1.6
  circle A18 centre (194.523733, 37.500003) radius 1.6
  line L66 (18.523733, 115.500002) -> (18.523733, 105.500002)
  line L67 (18.523733, 105.500002) -> (-26.476267, 105.500002)
  line L68 (-26.476267, 105.500002) -> (-26.476267, 115.500002)
  line L69 (-26.476267, 115.500002) -> (18.523733, 115.500002)
  line L70 (18.523733, 26.500002) -> (18.523733, 16.500002)
  line L71 (18.523733, 16.500002) -> (-26.476267, 16.500002)
  line L72 (-26.476267, 16.500002) -> (-26.476267, 26.500002)
  line L73 (-26.476267, 26.500002) -> (18.523733, 26.500002)
  circle A19 centre (0, -28.249998) radius 1.75
  circle A20 centre (0, 160.250001) radius 1.75
  circle A21 centre (195.047467, 160.250001) radius 1.75
  circle A22 centre (195.047467, -28.249997) radius 1.75
  circle A23 centre (177.047467, 160.250001) radius 1.75
  circle A24 centre (-18, 160.250001) radius 1.75
  circle A25 centre (-18, -28.249997) radius 1.75
  circle A26 centre (18, 160.250001) radius 1.75
  circle A27 centre (159.047467, -28.249998) radius 1.75
  circle A28 centre (177.047467, -28.249998) radius 1.75
  circle A29 centre (159.047467, 160.250001) radius 1.75
  circle A30 centre (18, -28.249998) radius 1.75
  circle A31 centre (53.523733, 156.000002) radius 5
  circle A32 centre (53.523733, -23.999998) radius 5
  line L74 (66.023733, 157.500002) -> (111.023733, 157.500002)
  line L75 (111.023733, 157.500002) -> (111.023733, -25.499998)
  line L76 (111.023733, -25.499998) -> (66.023733, -25.499998)
  line L77 (66.023733, -25.499998) -> (66.023733, 157.500002)
  line L78 (204.523733, 93.576493) -> (216.523733, 93.576493)
  line L79 (216.523733, 93.576493) -> (216.523733, 38.576493)
  line L80 (216.523733, 38.576493) -> (204.523733, 38.576493)
  line L81 (204.523733, 38.576493) -> (204.523733, 93.576493)
  circle A33 centre (-43.476267, 18.5) radius 1.75
  circle A34 centre (-43.476267, 55.625003) radius 1.75
  circle A35 centre (-43.476267, 113.500003) radius 1.75
  circle A36 centre (-43.476267, 76.375003) radius 1.75
  arc A37 (-38.476267, 163.500003) -> (-46.476267, 155.500003) centre (-38.476267, 155.500003) ccw
  line L82 (-46.476267, 155.500003) -> (-46.476267, 143.500003)
  line L83 (-46.476267, 143.500003) -> (-40.476267, 143.500003)
  line L84 (-40.476267, 143.500003) -> (-40.476267, 123.500003)
  line L85 (-40.476267, 123.500003) -> (-46.476267, 123.500003)
  line L86 (-46.476267, 123.500003) -> (-46.476267, 103.500003)
  line L87 (-46.476267, 103.500003) -> (-40.476267, 103.500003)
  line L88 (-40.476267, 103.500003) -> (-40.476267, 83.500003)
  line L89 (-40.476267, 83.500003) -> (-46.476267, 83.500003)
  line L90 (-46.476267, 83.500003) -> (-46.476267, 48.5)
  line L91 (-46.476267, 48.5) -> (-40.476267, 48.5)
  line L92 (-40.476267, 48.5) -> (-40.476267, 28.5)
  line L93 (-40.476267, 28.5) -> (-46.476267, 28.5)
  line L94 (-46.476267, 28.5) -> (-46.476267, 8.5)
  line L95 (-46.476267, 8.5) -> (-40.476267, 8.5)
  line L96 (-40.476267, 8.5) -> (-40.476267, -11.5)
  line L97 (-40.476267, -11.5) -> (-46.476267, -11.5)
  line L98 (-46.476267, -11.5) -> (-46.476267, -23.499997)
  arc A38 (-46.476267, -23.499997) -> (-38.476267, -31.499997) centre (-38.476267, -23.499997) ccw
  line L99 (-38.476267, -31.499997) -> (26.000003, -31.499999)
  arc A39 (30.000003, -35.5) -> (26.000003, -31.499999) centre (22.7085, -38.791502) ccw
  line L100 (30.000003, -35.5) -> (30.000003, -39)
  arc A40 (30.000003, -39) -> (38.000003, -47) centre (38.000003, -39) ccw
  line L101 (38.000003, -47) -> (138.802962, -47)
  arc A41 (138.802962, -47) -> (146.802962, -39) centre (138.802962, -39) ccw
  line L102 (146.802962, -39) -> (146.802962, -35.499999)
  arc A42 (150.802962, -31.499999) -> (146.802962, -35.499999) centre (154.094465, -38.791502) ccw
  line L103 (150.802962, -31.499999) -> (215.523733, -31.499997)
  arc A43 (215.523733, -31.499997) -> (223.523733, -23.499997) centre (215.523733, -23.499997) ccw
  line L104 (223.523733, -23.499997) -> (223.523733, 155.500003)
  arc A44 (223.523733, 155.500003) -> (215.523733, 163.500003) centre (215.523733, 155.500003) ccw
  line L105 (215.523733, 163.500003) -> (150.802962, 163.500003)
  arc A45 (146.802962, 167.770131) -> (150.802962, 163.500003) centre (154.237087, 170.72543) ccw
  line L106 (146.802962, 167.770131) -> (146.802961, 171.270131)
  arc A46 (146.802961, 171.270131) -> (138.802961, 179.270131) centre (138.802961, 171.270131) ccw
  line L107 (138.802961, 179.270131) -> (38.270127, 179.270131)
  arc A47 (38.270127, 179.270131) -> (30.270127, 171.270131) centre (38.270127, 171.270131) ccw
  line L108 (30.270127, 171.270131) -> (30.270127, 167.770131)
  arc A48 (26, 163.500003) -> (30.270127, 167.770131) centre (22.8966, 170.873531) ccw
  line L109 (26, 163.500003) -> (-38.476267, 163.500003)
  circle A49 centre (111.023733, -35.499998) radius 2
  circle A50 centre (88.523733, -35.499998) radius 2
  circle A51 centre (66.023733, -35.499998) radius 2
  circle A52 centre (111.023733, 167.500002) radius 2
  circle A53 centre (88.523733, 167.500002) radius 2
  circle A54 centre (66.023733, 167.500002) radius 2
  point P0 (553.278877, -1.422232)
  point P1 (135.336738, -1.986996)
  point P2 (38.773733, 66.100003)
  point P3 (-19.726267, 65.900003)
  point P4 (21.273733, 65.900003)
  point P5 (-2.226267, 66.100003)
  constraints: 2 other
extrude "Выдавливание18" cut sketch "Эскиз19" against normal blind 8 contours L0 L3 L2 L1 | A0 | L4 L7 L6 L5 | L9 L12 L11 L10 | A1 | L13 L14 L15 L16 | L17 L21 L20 L19 L18 | L22 L25 L24 L23 | A2 | L26 L27 L29 L28 | A4 A3 | A3 A4 | L46 L47 L48 L49 picked at (138.323354, 122.543257) picked at (137.847995, 124.810546)
